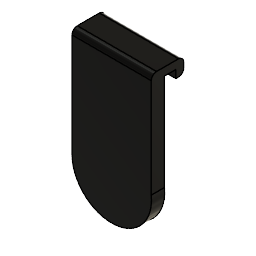
Tapas_Rodamientos (Autodesk Fusion 360 design; units mm, degrees)
Autodesk Fusion 360 part; units mm, degrees
sketch "Boceto1" plane through (0, 0, 0) normal (0, 1, 0) x (1, 0, 0)
  circle A0 centre (0, 0) radius 11
  circle A1 centre (0, 0) radius 12
  circle A2 centre (0, 0) radius 15
  line L0 (0, 0) -> (0, -0.3305)
  dimension "d1" = 22
  dimension "d2" = 1
  dimension "d3" = 30
  constraint coincident A0.centre A1.centre
  constraint concentric A0 A2
  constraint vertical L0
  measures "d1" diameter of A0
  measures "d3" diameter of A2
extrude "Extruir1" add sketch "Boceto1" against normal blind 1 contours A2 makes body 1
sketch "Boceto2" plane through (0, -1, 0) normal (0, -1, 0) x (1, 0, 0)
  circle A0 centre (0, 0) radius 12
  circle A1 centre (0, 0) radius 15
  circle A2 centre (0, 0) radius 6.075
  line L0 (-4.3795, 5.4797) -> (-6.9353, -1.0529)
  line L1 (-6.9353, -1.0529) -> (-2.5558, -6.5326)
  line L2 (-2.5558, -6.5326) -> (4.3795, -5.4797)
  line L3 (4.3795, -5.4797) -> (6.9353, 1.0529)
  line L4 (6.9353, 1.0529) -> (2.5558, 6.5326)
  line L5 (2.5558, 6.5326) -> (-4.3795, 5.4797)
  dimension "d6" = 12.15
  constraint concentric A0 A2
  constraint coincident A0.centre A1.centre
  measures "d6" diameter of A2
extrude "Extruir2" add sketch "Boceto2" along normal blind 5 contours A0 | A1 bodies 1
sketch "Boceto3" plane through (0, -6, 0) normal (0, -1, 0) x (1, 0, 0)
  circle A0 centre (0, 0) radius 15
  line L0 (-4.3795, 5.4797) -> (2.5558, 6.5326)
  line L1 (2.5558, 6.5326) -> (6.9353, 1.0529)
  line L2 (6.9353, 1.0529) -> (4.3795, -5.4797)
  line L3 (4.3795, -5.4797) -> (-2.5558, -6.5326)
  line L4 (-2.5558, -6.5326) -> (-6.9353, -1.0529)
  line L5 (-6.9353, -1.0529) -> (-4.3795, 5.4797)
extrude "Extruir3" add sketch "Boceto3" against normal blind 1 contours L0 L1 L2 L3 L4 L5 bodies 1
sketch "Boceto4" plane through (0, -5, 0) normal (0, 1, 0) x (-1, 0, 0)
  circle A0 centre (0, 0) radius 6
  line L0 (-0.4187, 6.9155) -> (-6.1984, 3.0951)
  line L1 (-6.1984, 3.0951) -> (-5.7797, -3.8204)
  line L2 (-5.7797, -3.8204) -> (0.4187, -6.9155)
  line L3 (0.4187, -6.9155) -> (6.1984, -3.0951)
  line L4 (6.1984, -3.0951) -> (5.7797, 3.8204)
  line L5 (5.7797, 3.8204) -> (-0.4187, 6.9155)
  line L6 (2.5558, -6.5326) -> (6.9353, -1.0529)
  line L7 (6.9353, -1.0529) -> (4.3795, 5.4797)
  line L8 (4.3795, 5.4797) -> (-2.5558, 6.5326)
  line L9 (-2.5558, 6.5326) -> (-6.9353, 1.0529)
  line L10 (-6.9353, 1.0529) -> (-4.3795, -5.4797)
  line L11 (-4.3795, -5.4797) -> (2.5558, -6.5326)
  dimension "d11" = 12
  constraint coincident A0.centre origin
  measures "d11" diameter of A0
extrude "Extruir4" add sketch "Boceto4" along normal blind 4 separate body contours A0 makes body 2
copy_body "Cuerpo - > Comp.1" bodies 1 removing the originals makes body 3 in component "Tapa Rodamiento"
copy_body "Cuerpo - > Comp.2" bodies 2 removing the originals makes body 4 in component "Imán 12x4mm"
extrude "Extruir1'" cut 1 faces at (13.8995, 0, 1.3414) along direction (0, -1, 0) up to surface (1 mm away) on bodies 3 bodies 3 in component "Tapa Rodamiento"
sketch "Boceto5" plane through (0, -1, 0) normal (0, 1, 0) x (-1, 0, 0)
  line L0 (-2.5558, 6.5326) -> (4.3795, 5.4797)
  line L1 (4.3795, 5.4797) -> (6.9353, -1.0529)
  line L2 (6.9353, -1.0529) -> (2.5558, -6.5326)
  line L3 (2.5558, -6.5326) -> (-4.3795, -5.4797)
  line L4 (-4.3795, -5.4797) -> (-6.9353, 1.0529)
  line L5 (-6.9353, 1.0529) -> (-2.5558, 6.5326)
  line L6 (0, 0) -> (-14.9161, 0)
  line L7 (0, 0) -> (0, 38)
  line L8 (-14.9161, 0) -> (15, 0)
  line L9 (15, 0) -> (15, 38)
  line L10 (15, 38) -> (-14.9161, 38)
  line L11 (-14.9161, 38) -> (-14.9161, 0)
  circle A0 centre (0, 0) radius 15
  dimension "d18" = 38
  constraint horizontal L6
  constraint perpendicular L6 L7
  constraint horizontal L8
  constraint vertical L9
  constraint horizontal L10
  constraint vertical L11
  measures "d18" distance of L6.start L7.end
extrude "Extruir2'" add sketch "Boceto5" against normal blind 5 contours L7 L10 L11 A0 | L7 L9 L10 A0 bodies 3 in component "Tapa Rodamiento"
sketch "Boceto6" plane through (14.9161, 0, 0) normal (1, 0, 0) x (0, 1, 0)
  line L0 (-1, 1.5845) -> (-1, 38)
  line L1 (-1, 38) -> (-6, 38)
  line L2 (-6, 38) -> (-6, 1.5845)
  line L3 (-6, 1.5845) -> (-1, 1.5845)
  line L4 (-6, 38) -> (-1, 38)
  line L5 (-1, 38) -> (-1, 41)
  line L6 (-1, 41) -> (-4, 41)
  line L7 (-6, 39) -> (-6, 38)
  line L8 (-1, 41) -> (3.3, 41)
  line L9 (3.3, 41) -> (3.3, 38)
  line L10 (3.3, 38) -> (-1, 38)
  line L11 (-1, 38) -> (-1, 41)
  line L12 (3.3, 41) -> (4.3, 41)
  line L13 (6.3, 39) -> (6.3, 37)
  line L14 (4.3, 35) -> (3.3, 35)
  line L15 (3.3, 35) -> (3.3, 41)
  arc A0 (4.3, 35) -> (6.3, 37) centre (4.3, 37) ccw
  arc A1 (6.3, 39) -> (4.3, 41) centre (4.3, 39) ccw
  arc A2 (-4, 41) -> (-6, 39) centre (-4, 39) ccw
  point P0 (6.3, 41)
  dimension "d21" = 4.3
  dimension "d22" = 3
  dimension "d23" = 2
  dimension "d24" = 2
  dimension "d25" = 2
  constraint horizontal L4
  constraint vertical L5
  constraint horizontal L6
  constraint vertical L7
  constraint coincident L1.end L2.start
  constraint horizontal L8
  constraint vertical L9
  constraint horizontal L10
  constraint vertical L11
  constraint horizontal L12
  constraint vertical L13
  constraint horizontal L14
  constraint vertical L15
  constraint tangent L13 A0
  constraint tangent L14 A0
  constraint coincident P0 L12
  constraint coincident P0 L13
  constraint tangent L12 A1
  constraint tangent L13 A1
  constraint tangent L6 A2
  constraint tangent L7 A2
  measures "d21" distance of L5.end L8.end
  measures "d22" distance of L8.end P0
  measures "d23" radius of A0
  measures "d24" radius of A1
  measures "d25" radius of A2
extrude "Extruir3'" add sketch "Boceto6" against normal up to surface (29.9161 mm away) contours L1 L4 L5 L6 L7 L11 A2 | L5 L8 L9 L10 L11 L15 | L9 L12 L13 L14 L15 A0 A1 bodies 3 in component "Tapa Rodamiento"
component "Tapa Rodamiento" placed x (1, 0, 0) y (0, 1, 0) z (0, 0, 1) at (0, 0, 0)
component "Imán 12x4mm" placed x (1, 0, 0) y (0, 1, 0) z (0, 0, 1) at (0, 0, 0)
named bodies: "Tapa Rodamiento", "Imán 12x4mm"
